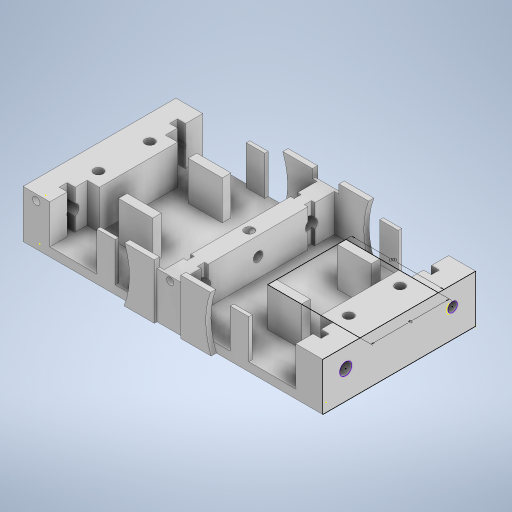
# Autodesk Inventor part: SCHOOL PROJECT
Saved by Autodesk Inventor 2024 (Build 280153000, 153)
## iProperties
Created: 2025-05-09
Part Number: SCHOOL PROJECT
Material: Generic
Document SubType Name: Modeling
Designer: arikm
Density: 1 g/cm^3
Appearance: Default
Author: arikm
Autodesk Inventor part; units mm, degrees
ref_plane "YZ Plane" through (0, 0, 0) normal (1, 0, 0) x (0, 1, 0)
ref_plane "XZ Plane" through (0, 0, 0) normal (0, 1, 0) x (-1, 0, 0)
ref_plane "XY Plane" through (0, 0, 0) normal (0, 0, 1) x (1, 0, 0)
sketch "Sketch1" plane through (0, 0, 0) normal (0, 1, 0) x (-1, 0, 0)
  line L0 (0, 0) -> (-70, 0)
  line L1 (-70, 0) -> (-70, -19.4)
  line L2 (-70, -19.4) -> (0, -19.4)
  line L3 (0, -19.4) -> (0, 0)
  line L4 (0, 0) -> (-4.4, 0)
  line L5 (-4.4, 0) -> (-4.4, -19.4)
  line L6 (-4.4, -19.4) -> (0, -19.4)
  line L7 (0, -19.4) -> (0, 0)
  line L8 (0, -9.7) -> (-4.4, -9.7)
  line L9 (0, -7.95) -> (-4.4, -7.95)
  line L10 (0, -11.45) -> (-4.4, -11.45)
  line L11 (5, -24.4) -> (-75, -24.4)
  line L12 (-75, -24.4) -> (-75, 5)
  line L13 (-75, 5) -> (5, 5)
  line L14 (5, 5) -> (5, -24.4)
  line L15 (-75, 0) -> (-75, 2)
  line L16 (-75, 2) -> (5, 2)
  dimension "d0" = 70
  dimension "d1" = 19.4
  dimension "d2" = 4.4
  dimension "d3" = 1.75
  dimension "d4" = 1.75
  dimension "d5" = 5
  dimension "d6" = 2
  constraints: 34 end point, 8 parallel, 4 perpendicular, 4 point on line, 2 horizontal, 2 midpoint, 3 other
  measures "d0" distance of L2.end L1.end
  measures "d1" distance of L1.end L0.end
  measures "d2" distance of L6.end L5.end
  measures "d3" distance between parallel lines of L8 L9
  measures "d4" distance between parallel lines of L8 L10
  measures "d5" distance between parallel lines of L2 L11
  measures "d6" distance of L15.start L15.end
extrude "Extrusion1" add sketch "Sketch1" along normal blind 22.4 contours L3 L9 L5 L0 | L3 L2 L5 L10 | L11 L12 L16 L14
sketch "Sketch2" plane through (0, 0, 0) normal (0, -1, 0) x (1, 0, 0)
  line L0 (-5, -24.4) -> (-5, 2) projected
  line L1 (75, -24.4) -> (-5, -24.4) projected
  line L2 (-5, 2) -> (75, 2)
  line L3 (75, 2) -> (75, -24.4)
  line L4 (75, -24.4) -> (-5, -24.4)
  line L5 (-5, -24.4) -> (-5, 2)
  point P0 (0, 0)
  constraints: 8 end point, 2 parallel, 1 horizontal, 1 perpendicular
extrude "Extrusion2" add sketch "Sketch2" along normal blind 1
sketch "Sketch3" plane through (0, 22.4, 0) normal (0, 1, 0) x (1, 0, 0)
  line L0 (75, -2) -> (75, 24.4) projected
  line L1 (75, 24.4) -> (48, 24.4)
  line L2 (48, 24.4) -> (48, -5.6)
  line L3 (48, -5.6) -> (75, -5.6)
  line L4 (75, -5.6) -> (75, 24.4)
  point P0 (0, 0)
  dimension "d11" = 27
  dimension "d12" = 30
  constraints: 8 end point, 2 parallel, 1 horizontal, 1 perpendicular
  measures "d11" distance of L3.end L2.end
  measures "d12" distance of L2.end L1.end
extrude "Extrusion3" cut sketch "Sketch3" against normal up to surface (22.4 mm away)
sketch "Sketch4" plane through (0, 22.4, 0) normal (0, 1, 0) x (1, 0, 0)
  line L0 (48, 0) -> (4.4, 0) projected
  line L1 (4.4, 0) -> (13.4, 0)
  line L2 (13.4, 0) -> (12.4, 0)
  line L3 (12.4, 0) -> (17.4, 0)
  line L4 (17.4, 0) -> (12.4, 0)
  line L5 (12.4, 0) -> (12.4, -8.176)
  line L6 (12.4, -8.176) -> (17.4, -8.176)
  line L7 (17.4, -8.176) -> (17.4, 0)
  line L8 (12.4, -8.176) -> (17.4, -8.176)
  line L9 (17.4, -8.176) -> (17.4, 29.1171)
  line L10 (17.4, 29.1171) -> (12.4, 29.1171)
  line L11 (12.4, 29.1171) -> (12.4, -8.176)
  point P0 (0, 0)
  dimension "d15" = 9
  dimension "d16" = 1
  dimension "d17" = 5
  constraints: 22 end point, 4 parallel, 4 point on line, 2 horizontal, 2 perpendicular
  measures "d15" distance of L0.end L1.end
  measures "d16" distance of L1.end L2.end
  measures "d17" distance of L2.end L3.end
extrude "Extrusion4" cut sketch "Sketch4" against normal up to surface (22.4 mm away)
sketch "Sketch5" plane through (-5, -1, 2) normal (0, 0, 1) x (1, 0, 0)
  line L0 (17.4, 1) -> (22.4, 1) projected
  line L1 (53, 23.4) -> (22.4, 23.4) projected
  line L2 (17.4, 1) -> (27.4, 1)
  line L3 (27.4, 1) -> (27.4, 23.4)
  line L4 (27.4, 23.4) -> (17.4, 23.4)
  line L5 (17.4, 23.4) -> (17.4, 1)
  point P0 (5, 1)
  dimension "d20" = 10
  constraints: 8 end point, 2 parallel, 1 horizontal, 1 perpendicular, 1 point on line
  measures "d20" distance of L4.end L3.end
extrude "Extrusion5" cut sketch "Sketch5" against normal through all
sketch "Sketch6" plane through (-5, -1, 2) normal (0, 0, 1) x (1, 0, 0)
  line L0 (17.4, 23.4) -> (17.4, 1) projected
  line L1 (17.4, 23.4) -> (9.4, 23.4)
  line L2 (17.4, 23.4) -> (0, 23.4) projected
  line L3 (53, 23.4) -> (27.4, 23.4) projected
  line L4 (27.4, 23.4) -> (35.4, 23.4)
  line L5 (9.4, 23.4) -> (35.4, 23.4)
  line L6 (35.4, 23.4) -> (35.4, 1)
  line L7 (35.4, 1) -> (9.4, 1)
  line L8 (9.4, 1) -> (9.4, 23.4)
  point P0 (5, 1)
  dimension "d23" = 8
  dimension "d24" = 8
  constraints: 12 end point, 2 parallel, 2 point on line, 1 horizontal, 1 perpendicular
  measures "d23" distance of L0.start L1.end
  measures "d24" distance of L3.end L4.end
extrude "Extrusion6" cut sketch "Sketch6" against normal blind 10
sketch "Sketch7" plane through (0, 0, 0) normal (0, 1, 0) x (1, 0, 0)
  line L0 (-5, 24.4) -> (75, 24.4) projected
  line L1 (75, 24.4) -> (75, 59.4)
  line L2 (75, -2) -> (-5, -2) projected
  line L3 (75, -2) -> (-5, -2)
  line L4 (-5, -2) -> (-5, 24.4)
  line L5 (-5, 24.4) -> (75, 24.4)
  line L6 (75, 24.4) -> (75, -2)
  line L7 (4.4, -2) -> (4.4, 7.95) projected
  line L8 (4.4, 7.95) -> (4.4, -2)
  line L9 (4.4, 7.95) -> (0, 7.95)
  line L10 (0, 7.95) -> (0, 11.45) projected
  line L11 (0, 7.95) -> (0, 11.45)
  line L12 (0, 11.45) -> (4.4, 11.45)
  line L13 (4.4, 11.45) -> (4.4, 19.4) projected
  line L14 (0, 11.45) -> (4.4, 11.45)
  line L15 (4.4, 11.45) -> (4.4, 19.4)
  line L16 (12.4, 19.4) -> (12.4, 24.4) projected
  line L17 (4.4, 19.4) -> (12.4, 19.4)
  line L18 (12.4, 19.4) -> (12.4, 24.4)
  line L19 (22.4, 19.4) -> (22.4, 24.4) projected
  line L20 (12.4, 24.4) -> (22.4, 24.4)
  line L21 (22.4, 19.4) -> (48, 19.4) projected
  line L22 (22.4, 24.4) -> (48, 24.4)
  line L23 (48, 24.4) -> (48, 19.4)
  line L24 (48, 19.4) -> (22.4, 19.4)
  line L25 (22.4, 19.4) -> (22.4, 24.4)
  line L26 (75, 41.9) -> (-5, 41.9)
  line L27 (48, 0) -> (30.4, 0) projected
  line L28 (30.4, -2) -> (48, -2)
  line L29 (48, -2) -> (48, 0)
  line L30 (48, 0) -> (30.4, 0)
  line L31 (30.4, 0) -> (30.4, -2)
  line L32 (-5, 59.4) -> (75, 59.4)
  line L33 (75, 85.8) -> (-5, 85.8)
  line L34 (-5, 85.8) -> (-5, 59.4)
  line L35 (75, 59.4) -> (75, 85.8)
  line L36 (4.4, 75.85) -> (4.4, 85.8)
  line L37 (4.4, 75.85) -> (0, 75.85)
  line L38 (0, 75.85) -> (0, 72.35)
  line L39 (0, 72.35) -> (4.4, 72.35)
  line L40 (4.4, 72.35) -> (4.4, 64.4)
  line L41 (12.4, 64.4) -> (12.4, 59.4)
  line L42 (4.4, 64.4) -> (12.4, 64.4)
  line L43 (22.4, 64.4) -> (22.4, 59.4)
  line L44 (48, 59.4) -> (48, 64.4)
  line L45 (48, 64.4) -> (22.4, 64.4)
  line L46 (48, 83.8) -> (30.4, 83.8)
  line L47 (48, 85.8) -> (48, 83.8)
  line L48 (30.4, 83.8) -> (30.4, 85.8)
  point P0 (0, 0)
  dimension "d27" = 35
  constraints: 80 end point, 24 symmetric about line, 7 perpendicular, 6 parallel, 5 horizontal, 4 collinear, 1 midpoint, 1 point on line, 1 vertical
  measures "d27" distance of L0.end L1.end
extrude "Extrusion7" add sketch "Sketch7" against normal blind 1 contours L34 L33 L36 L37 L38 L39 L40 L42 L41 L32 | L41 L42 L40 L39 L38 L37 L36 L33 L48 L46 L47 L35 L32 L44 L45 L43 | L43 L45 L44 L32 | L33 L47 L46 L48
extrude "Extrusion8" add sketch "Sketch7" along normal up to surface (22.4 mm away) contours L34 L33 L36 L37 L38 L39 L40 L42 L41 L32 | L43 L45 L44 L32 | L33 L47 L46 L48
thicken "Thicken1" operation cut thickness 1 both sides no extend neighbours no toward (1, 0, 0) faces at (30.4, 7.4667, 0.6667)
thicken "Thicken2" operation cut thickness 1 both sides no extend neighbours no toward (1, 0, 0) faces at (30.4, 7.4667, -85.1333)
thicken "Thicken3" operation cut thickness 1 both sides no extend neighbours no toward (-1, 0, 0) faces at (12.4, 7.4667, -22.7333)
thicken "Thicken4" operation cut thickness 1 both sides no extend neighbours no toward (-1, 0, 0) faces at (12.4, 7.4667, -61.0667)
thicken "Thicken7" operation cut thickness 0.2 both sides no extend neighbours no toward (-1, 0, 0) faces at (0, 7.4667, -9.1167)
thicken "Thicken8" operation cut thickness 0.2 both sides no extend neighbours no toward (-1, 0, 0) faces at (0, 7.4667, -73.5167)
sketch "Sketch8" plane through (0, 22.4, 0) normal (0, 1, 0) x (1, 0, 0)
  line L0 (48, 0) -> (48, -2) projected
  line L1 (-5, 85.8) -> (75, 85.8) projected
  line L2 (48, -2) -> (42, -2)
  line L3 (42, -2) -> (42, 85.8)
  line L4 (42, 85.8) -> (48, 85.8)
  line L5 (48, 85.8) -> (48, -2)
  point P0 (0, 0)
  dimension "d48" = 6
  constraints: 8 end point, 2 parallel, 1 horizontal, 1 perpendicular, 1 point on line
  measures "d48" distance of L3.end L4.end
extrude "Extrusion9" cut sketch "Sketch8" against normal up to surface (22.4 mm away)
sketch "Sketch9" plane through (0, 0, 0) normal (0, 1, 0) x (1, 0, 0)
  line L0 (75, 24.4) -> (75, -2) projected
  line L1 (-5, 24.4) -> (75, 24.4) projected
  line L2 (75, -2) -> (70, -2)
  line L3 (70, -2) -> (70, 24.4)
  line L4 (70, 24.4) -> (75, 24.4)
  line L5 (75, 24.4) -> (75, -2)
  line L6 (75, 59.4) -> (75, 85.8) projected
  line L7 (-5, 85.8) -> (75, 85.8) projected
  line L8 (75, 59.4) -> (70, 59.4)
  line L9 (70, 59.4) -> (70, 85.8)
  line L10 (70, 85.8) -> (75, 85.8)
  line L11 (75, 85.8) -> (75, 59.4)
  point P0 (0, 0)
  dimension "d51" = 5
  dimension "d52" = 5
  constraints: 16 end point, 4 parallel, 2 horizontal, 2 perpendicular, 2 point on line
  measures "d51" distance of L3.end L4.end
  measures "d52" distance of L9.end L10.end
extrude "Extrusion10" add sketch "Sketch9" along normal up to surface (22.4 mm away)
sketch "Sketch10" plane through (75, -1, 2) normal (1, 0, 0) x (0, 0, -1)
  line L0 (2, 1) -> (0, 1) projected
  line L1 (26.4, 23.4) -> (26.4, 1) projected
  line L2 (0, 1) -> (26.4, 1)
  line L3 (26.4, 1) -> (26.4, 23.4)
  line L4 (26.4, 23.4) -> (0, 23.4)
  line L5 (0, 23.4) -> (0, 1)
  line L6 (0, 12.2) -> (87.8, 12.2)
  line L7 (87.8, 1) -> (87.8, 23.4) projected
  line L8 (61.4, 0) -> (61.4, 23.4) projected
  line L9 (61.4, 12.2) -> (87.8, 12.2)
  circle A0 centre (13.2, 12.2) radius 3.5
  circle A1 centre (74.6, 12.2) radius 3.5
  dimension "d55" = 7
  dimension "d56" = 7
  constraints: 12 end point, 3 midpoint, 3 point on line, 2 centre point, 2 parallel, 1 collinear, 1 horizontal, 1 perpendicular
  measures "d55" diameter of A0
  measures "d56" diameter of A1
extrude "Extrusion11" cut sketch "Sketch10" against normal through all contours A0 L6 | L6 A0 | A1 L6 | L6 A1
sketch "Sketch11" plane through (70, 22.4, 2) normal (0, 1, 0) x (1, 0, 0)
  line L0 (0, 0) -> (0, 26.4) projected
  line L1 (0, 13.2) -> (2, 13.2)
  line L2 (0, 13.2) -> (2, 13.2) construction
  line L3 (2, 13.2) -> (0, 13.2)
  line L4 (0, 13.2) -> (0, 11.2)
  line L5 (0, 11.2) -> (2, 11.2)
  line L6 (2, 11.2) -> (2, 13.2)
  line L7 (0, 11.2) -> (2, 11.2)
  line L8 (2, 11.2) -> (2, 15.2)
  line L9 (2, 15.2) -> (0, 15.2)
  line L10 (0, 15.2) -> (0, 11.2)
  line L11 (0, 61.4) -> (0, 87.8) projected
  line L12 (0, 74.6) -> (2, 74.6)
  line L13 (2, 74.6) -> (2, 73.4639)
  line L14 (2, 73.4639) -> (0, 73.4639)
  line L15 (0, 73.4639) -> (0, 74.6)
  line L16 (2, 74.6) -> (0, 74.6)
  line L17 (0, 74.6) -> (0, 76.6)
  line L18 (0, 76.6) -> (2, 76.6)
  line L19 (2, 76.6) -> (2, 74.6)
  line L20 (0, 74.6) -> (2, 74.6)
  line L21 (2, 74.6) -> (2, 72.6)
  line L22 (2, 72.6) -> (0, 72.6)
  line L23 (0, 72.6) -> (0, 74.6)
  point P0 (-70, 2)
  point P1 (2, 13.2)
  point P2 (0, 15.2)
  point P3 (2, 73.4639)
  dimension "d59" = 2
  dimension "d60" = 0
  dimension "d61" = 2
  dimension "d62" = 4
  dimension "d63" = 2
  dimension "d64" = 2
  dimension "d65" = 2
  constraints: 44 end point, 10 parallel, 7 horizontal, 5 perpendicular, 4 point on line, 2 midpoint, 1 collinear
  measures "d59" distance of L1.start L1.end
  measures "d60" distance between parallel lines of L1 L2
  measures "d61" distance of L4.end L3.end
  measures "d62" distance of L8.end L7.end
  measures "d63" distance of L13.end L14.end
  measures "d64" distance of L16.end L17.end
  measures "d65" distance of L20.end L21.end
extrude "Extrusion12" cut sketch "Sketch11" against normal up to surface contours L0 L1 L6 L5 | L0 L9 L8 L1 round surface about axis through (75, 11.2, -11.2) along (-1, 0, 0) radius 3.5 far side no
extrude "Extrusion13" cut sketch "Sketch11" against normal up to surface contours L11 L14 L21 L22 | L11 L12 L13 L14 | L11 L18 L19 L12 round surface about axis through (75, 11.2, -72.6) along (-1, 0, 0) radius 3.5 far side no
sketch "Sketch12" plane through (0, 22.4, 0) normal (0, 1, 0) x (1, 0, 0)
  line L0 (4.4, 14.7) -> (4.4, 11.45) projected
  line L1 (-0.2, 11.45) -> (4.4, 11.45)
  line L2 (4.4, 11.45) -> (4.4, 12.45)
  line L3 (4.4, 12.45) -> (-0.2, 12.45)
  line L4 (-0.2, 12.45) -> (-0.2, 11.45)
  point P0 (0, 0)
  dimension "d70" = 1
  constraints: 8 end point, 2 parallel, 1 horizontal, 1 perpendicular, 1 point on line
  measures "d70" distance of L2.end L1.end
extrude "Extrusion14" cut sketch "Sketch12" against normal up to surface (22.4 mm away)
sketch "Sketch13" plane through (-5, 22.4, -85.8) normal (0, 1, 0) x (1, 0, 0)
  line L0 (9.4, -13.45) -> (9.4, -21.4) projected
  line L1 (9.4, -13.45) -> (4.8, -13.45)
  line L2 (4.8, -13.45) -> (4.8, -14.45)
  line L3 (4.8, -14.45) -> (9.4, -14.45)
  line L4 (9.4, -14.45) -> (9.4, -13.45)
  point P0 (5, -85.8)
  point P1 (9.4, -14.45)
  dimension "d73" = 1
  constraints: 8 end point, 2 parallel, 1 horizontal, 1 perpendicular
  measures "d73" distance of L2.end L1.end
extrude "Extrusion15" cut sketch "Sketch13" against normal up to surface (22.4 mm away)
sketch "Sketch14" plane through (0, 0, 0) normal (0, 1, 0) x (1, 0, 0)
  line L0 (11.4, 24.4) -> (-5, 24.4) projected
  line L1 (75, 59.4) -> (-5, 59.4) projected
  line L2 (-5, 24.4) -> (75, 24.4)
  line L3 (75, 24.4) -> (75, 59.4)
  line L4 (75, 59.4) -> (-5, 59.4)
  line L5 (-5, 59.4) -> (-5, 24.4)
  point P0 (0, 0)
  constraints: 8 end point, 2 parallel, 1 horizontal, 1 perpendicular
extrude "Extrusion16" add sketch "Sketch14" against normal up to surface (1 mm away)
sketch "Sketch15" plane through (0, 0, 0) normal (0, 1, 0) x (1, 0, 0)
  line L0 (-5, -2) -> (-5, 85.8) projected
  line L1 (75, 85.8) -> (75, -2) projected
  line L2 (-5, -2) -> (75, -2)
  line L3 (75, -2) -> (75, 85.8)
  line L4 (75, 85.8) -> (-5, 85.8)
  line L5 (-5, 85.8) -> (-5, -2)
  line L6 (-0.2, 7.95) -> (-0.2, 12.45) projected
  line L7 (-0.2, 12.45) -> (4.4, 12.45) projected
  line L8 (-0.2, 7.95) -> (4.4, 7.95)
  line L9 (4.4, 7.95) -> (4.4, 12.45)
  line L10 (4.4, 12.45) -> (-0.2, 12.45)
  line L11 (-0.2, 12.45) -> (-0.2, 7.95)
  line L12 (11.4, 24.4) -> (-5, 24.4) projected
  line L13 (4.4, 19.4) -> (11.4, 19.4) projected
  line L14 (-5, 24.4) -> (11.4, 24.4)
  line L15 (11.4, 24.4) -> (11.4, 19.4)
  line L16 (11.4, 19.4) -> (-5, 19.4)
  line L17 (-5, 19.4) -> (-5, 24.4)
  line L18 (-5, -2) -> (4.4, -2)
  line L19 (4.4, -2) -> (4.4, 19.4)
  line L20 (4.4, 19.4) -> (-5, 19.4)
  line L21 (-5, 19.4) -> (-5, -2)
  line L22 (11.4, 19.4) -> (-5, 19.4)
  line L23 (-5, 19.4) -> (-5, 24.4)
  line L24 (-5, 24.4) -> (11.4, 24.4)
  line L25 (11.4, 24.4) -> (11.4, 19.4)
  line L26 (31.4, -2) -> (31.4, 0) projected
  line L27 (42, 0) -> (31.4, 0) projected
  line L28 (31.4, -2) -> (42, -2)
  line L29 (42, -2) -> (42, 0)
  line L30 (42, 0) -> (31.4, 0)
  line L31 (31.4, 0) -> (31.4, -2)
  line L32 (22.4, 24.4) -> (22.4, 19.4) projected
  line L33 (22.4, 19.4) -> (42, 19.4)
  line L34 (42, 19.4) -> (42, 24.4)
  line L35 (42, 24.4) -> (22.4, 24.4)
  line L36 (22.4, 24.4) -> (22.4, 19.4)
  line L37 (70, 13.2) -> (70, 24.4) projected
  line L38 (75, -2) -> (70, -2)
  line L39 (70, -2) -> (70, 24.4)
  line L40 (70, 24.4) -> (75, 24.4)
  line L41 (75, 24.4) -> (75, -2)
  line L42 (70, 9.2) -> (72, 9.2) projected
  line L43 (72, 13.2) -> (70, 13.2) projected
  line L44 (70, 9.2) -> (72, 9.2)
  line L45 (72, 9.2) -> (72, 13.2)
  line L46 (72, 13.2) -> (70, 13.2)
  line L47 (70, 13.2) -> (70, 9.2)
  line L48 (-5, 59.4) -> (-5, 24.4) projected
  line L49 (-5, 41.9) -> (75, 41.9)
  line L50 (-5, 85.8) -> (-5, -2)
  line L51 (75, -2) -> (75, 85.8)
  line L52 (-5, 85.8) -> (75, 85.8)
  line L53 (-0.2, 75.85) -> (-0.2, 71.35)
  line L54 (-0.2, 71.35) -> (4.4, 71.35)
  line L55 (-0.2, 75.85) -> (4.4, 75.85)
  line L56 (4.4, 75.85) -> (4.4, 71.35)
  line L57 (4.4, 64.4) -> (11.4, 64.4)
  line L58 (-5, 59.4) -> (11.4, 59.4)
  line L59 (4.4, 85.8) -> (4.4, 64.4)
  line L60 (11.4, 59.4) -> (11.4, 64.4)
  line L61 (31.4, 85.8) -> (31.4, 83.8)
  line L62 (42, 83.8) -> (31.4, 83.8)
  line L63 (42, 85.8) -> (42, 83.8)
  line L64 (70, 85.8) -> (70, 59.4)
  line L65 (70, 59.4) -> (75, 59.4)
  line L66 (70, 74.6) -> (72, 74.6)
  line L67 (72, 70.6) -> (70, 70.6)
  line L68 (72, 74.6) -> (72, 70.6)
  line L69 (155, -2) -> (155, 85.8)
  line L70 (155, -2) -> (75, -2)
  line L71 (75, 85.8) -> (155, 85.8)
  line L72 (150.2, 7.95) -> (150.2, 12.45)
  line L73 (150.2, 12.45) -> (145.6, 12.45)
  line L74 (150.2, 7.95) -> (145.6, 7.95)
  line L75 (138.6, 24.4) -> (155, 24.4)
  line L76 (145.6, 19.4) -> (138.6, 19.4)
  line L77 (138.6, 24.4) -> (138.6, 19.4)
  line L78 (145.6, -2) -> (145.6, 19.4)
  line L79 (155, 19.4) -> (155, -2)
  line L80 (118.6, -2) -> (118.6, 0)
  line L81 (108, -2) -> (108, 0)
  line L82 (108, 0) -> (118.6, 0)
  line L83 (127.6, 24.4) -> (127.6, 19.4)
  line L84 (127.6, 19.4) -> (108, 19.4)
  line L85 (108, 19.4) -> (108, 24.4)
  line L86 (108, 24.4) -> (127.6, 24.4)
  line L87 (80, -2) -> (80, 24.4)
  line L88 (80, 24.4) -> (75, 24.4)
  line L89 (80, 9.2) -> (78, 9.2)
  line L90 (78, 13.2) -> (80, 13.2)
  line L91 (78, 9.2) -> (78, 13.2)
  line L92 (150.2, 75.85) -> (145.6, 75.85)
  line L93 (150.2, 75.85) -> (150.2, 71.35)
  line L94 (150.2, 71.35) -> (145.6, 71.35)
  line L95 (145.6, 75.85) -> (145.6, 71.35)
  line L96 (145.6, 85.8) -> (145.6, 64.4)
  line L97 (155, 59.4) -> (138.6, 59.4)
  line L98 (138.6, 59.4) -> (138.6, 64.4)
  line L99 (145.6, 64.4) -> (138.6, 64.4)
  line L100 (108, 83.8) -> (118.6, 83.8)
  line L101 (108, 85.8) -> (108, 83.8)
  line L102 (118.6, 85.8) -> (118.6, 83.8)
  line L103 (80, 85.8) -> (80, 59.4)
  line L104 (80, 59.4) -> (75, 59.4)
  line L105 (78, 74.6) -> (78, 70.6)
  line L106 (80, 74.6) -> (78, 74.6)
  line L107 (78, 70.6) -> (80, 70.6)
  line L108 (155, 41.9) -> (75, 41.9)
  line L109 (127.6, 19.4) -> (108, 19.4)
  line L110 (108, 19.4) -> (108, 24.4)
  line L111 (108, 24.4) -> (127.6, 24.4)
  line L112 (127.6, 24.4) -> (127.6, 19.4)
  line L113 (127.6, 19.4) -> (108, 19.4)
  line L114 (108, 19.4) -> (108, 24.4)
  line L115 (108, 24.4) -> (127.6, 24.4)
  line L116 (127.6, 24.4) -> (127.6, 19.4)
  line L117 (108, 64.4) -> (108, 59.4)
  line L118 (127.6, 64.4) -> (108, 64.4)
  line L119 (127.6, 59.4) -> (127.6, 64.4)
  line L120 (108, 59.4) -> (127.6, 59.4)
  point P0 (0, 0)
  point P1 (75, -2)
  constraints: 216 end point, 86 symmetric about line, 22 parallel, 12 horizontal, 11 perpendicular, 4 point on line, 3 midpoint
extrude "Extrusion17" add sketch "Sketch15" against normal blind 1 contours L108 L69 L75 L77 L76 L78 L70 L80 L82 L81 L87 L88 L1 | L1 L104 L103 L71 L101 L100 L102 L96 L95 L99 L98 L97 L69 L108 | L1 L71 L103 L106 L105 L107 L104 | L88 L87 L90 L91 L89 L70 L1 | L69 L70 L78 L74 L72 L73 L76 L77 L75 | L97 L98 L99 L96 L94 L93 L92 L71 L69 | L107 L105 L106 L103 | L87 L89 L91 L90 | L81 L82 L80 L70 | L71 L102 L100 L101 | L92 L93 L94 L95 | L78 L73 L72 L74 | L83 L84 L85 L86 | L118 L119 L120 L117
extrude "Extrusion18" add sketch "Sketch15" along normal up to surface (22.4 mm away) contours L1 L71 L103 L106 L105 L107 L104 | L88 L87 L90 L91 L89 L70 L1 | L69 L70 L78 L74 L72 L73 L76 L77 L75 | L97 L98 L99 L96 L94 L93 L92 L71 L69 | L81 L82 L80 L70 | L71 L102 L100 L101 | L83 L84 L85 L86 | L118 L119 L120 L117
sketch "Sketch16" plane through (-5, 22.4, -24.4) normal (-1, 0, 0) x (0, 0, 1)
  arc A0 (-51.45, -9.901) -> (-51.45, -12.499) centre (-48.2, -11.2) ccw projected
  circle A1 centre (-48.2, -11.2) radius 3.5
  circle A2 centre (13.2, -11.2) radius 3.5 projected
  circle A3 centre (13.2, -11.2) radius 3.5
  point P0 (24.4, -22.4)
  constraints: 2 centre point, 2 coincident
extrude "Extrusion19" add sketch "Sketch16" against normal through all
extrude "Extrusion20" cut sketch "Sketch16" against normal through all
sketch "Sketch17" plane through (0, -1, 0) normal (0, -1, 0) x (1, 0, 0)
  line L0 (-5, -85.8) -> (155, -85.8) projected
  line L1 (155, 2) -> (-5, 2)
  line L2 (-5, 2) -> (-5, -85.8)
  line L3 (-5, -85.8) -> (155, -85.8)
  line L4 (155, -85.8) -> (155, 2)
  point P0 (0, 0)
  constraints: 8 end point, 2 parallel, 1 horizontal, 1 perpendicular
extrude "Extrusion21" add sketch "Sketch17" along normal blind 4
sketch "Sketch18" plane through (0, 0, 0) normal (0, 1, 0) x (1, 0, 0)
  line L0 (22.4, 59.4) -> (42, 59.4) projected
  line L1 (32.2, 59.4) -> (32.2, 24.4)
  line L2 (42, 24.4) -> (22.4, 24.4) projected
  line L3 (108, 24.4) -> (127.6, 24.4) projected
  line L4 (117.8, 24.4) -> (117.8, 59.4)
  line L5 (127.6, 59.4) -> (108, 59.4) projected
  line L6 (80, 24.4) -> (70, 24.4) projected
  line L7 (75, 24.4) -> (75, 59.4)
  line L8 (80, 59.4) -> (70, 59.4) projected
  circle A0 centre (32.2, 41.9) radius 3.25
  circle A1 centre (75, 41.9) radius 3.25
  circle A2 centre (117.8, 41.9) radius 3.25
  point P0 (0, 0)
  dimension "d88" = 6.5
  dimension "d89" = 6.5
  dimension "d90" = 6.5
  constraints: 9 midpoint, 6 end point, 3 centre point
  measures "d88" diameter of A0
  measures "d89" diameter of A1
  measures "d90" diameter of A2
extrude "Extrusion22" cut sketch "Sketch18" against normal through all
sketch "Sketch19" plane through (0, 0, 0) normal (0, 1, 0) x (1, 0, 0)
  circle A0 centre (32.2, 41.9) radius 3.25 projected
  circle A1 centre (32.2, 41.9) radius 5
  circle A2 centre (75, 41.9) radius 3.25 projected
  circle A3 centre (75, 41.9) radius 5
  circle A4 centre (117.8, 41.9) radius 3.25 projected
  circle A5 centre (117.8, 41.9) radius 5
  point P0 (0, 0)
  dimension "d93" = 10
  dimension "d94" = 10
  dimension "d95" = 10
  constraints: 3 centre point, 3 coincident
  measures "d93" diameter of A1
  measures "d94" diameter of A3
  measures "d95" diameter of A5
extrude "Extrusion23" cut sketch "Sketch19" against normal blind 3 contours A0 | A1 | A2 | A3 | A4 | A5
sketch "Sketch20" plane through (0, 0, 0) normal (0, 1, 0) x (1, 0, 0)
  circle A0 centre (75, 41.9) radius 5 projected
  circle A1 centre (75, 41.9) radius 100
  line L0 (138.6, 24.4) -> (155, 24.4) projected
  line L1 (146.8, 24.4) -> (146.8, 59.4)
  line L2 (155, 59.4) -> (138.6, 59.4) projected
  line L3 (155, 59.4) -> (138.6, 59.4)
  line L4 (138.6, 59.4) -> (138.6, 24.4)
  line L5 (138.6, 24.4) -> (155, 24.4)
  line L6 (155, 24.4) -> (155, 59.4)
  line L7 (-5, -2) -> (-5, 85.8) projected
  line L8 (11.4, 64.4) -> (11.4, 59.4) projected
  line L9 (-5, 24.4) -> (11.4, 24.4)
  line L10 (11.4, 24.4) -> (11.4, 59.4)
  line L11 (11.4, 59.4) -> (-5, 59.4)
  line L12 (-5, 59.4) -> (-5, 24.4)
  point P0 (0, 0)
  constraints: 18 end point, 4 parallel, 2 horizontal, 2 midpoint, 2 perpendicular, 1 centre point, 1 coincident, 1 point on line
extrude "Extrusion24" add sketch "Sketch20" along normal up to surface (22.4 mm away) contours L4 L2 L1 L0 | L1 L2 L6 L0 | L7 L11 L10 L9
sketch "Sketch21" plane through (0, 0, 0) normal (0, 1, 0) x (1, 0, 0)
  line L0 (67.8253, 32.1607) -> (82.8688, 32.1607)
  line L1 (82.8688, 32.1607) -> (82.8688, 49.81)
  line L2 (82.8688, 49.81) -> (67.8253, 49.81)
  line L3 (67.8253, 49.81) -> (67.8253, 32.1607)
  point P0 (0, 0)
  constraints: 8 end point, 2 parallel, 1 horizontal, 1 perpendicular
extrude "Extrusion25" add sketch "Sketch21" against normal up to surface (5 mm away)
sketch "Sketch22" plane through (0, 0, 0) normal (0, 1, 0) x (1, 0, 0)
  line L0 (70, -2) -> (70, 24.4) projected
  line L1 (80, 70.6) -> (80, 59.4) projected
  line L2 (70, 24.4) -> (80, 24.4)
  line L3 (80, 24.4) -> (80, 59.4)
  line L4 (80, 59.4) -> (70, 59.4)
  line L5 (70, 59.4) -> (70, 24.4)
  point P0 (0, 0)
  constraints: 8 end point, 2 parallel, 1 horizontal, 1 perpendicular
extrude "Extrusion26" add sketch "Sketch22" along normal up to surface (22.4 mm away)
sketch "Sketch23" plane through (70, 22.4, 2) normal (0, 1, 0) x (1, 0, 0)
  line L0 (0, 15.2) -> (0, 72.6) projected
  line L1 (0, 43.9) -> (10, 43.9)
  line L2 (10, 72.6) -> (10, 15.2) projected
  circle A0 centre (5, 43.9) radius 2.7
  line L3 (68.7195, 43.9) -> (85, 43.9)
  line L4 (85, 87.8) -> (85, 0) projected
  line L5 (76.8598, 43.9) -> (76.8598, 14.45)
  line L6 (80.2, 14.45) -> (75.6, 14.45) projected
  line L7 (76.8598, 43.9) -> (76.8598, 73.35)
  line L8 (75.6, 73.35) -> (80.2, 73.35) projected
  line L9 (5, 43.9) -> (5, 33.1975)
  line L10 (-66.8598, 43.9) -> (-66.8598, 14.45)
  line L11 (-66.8598, 43.9) -> (-66.8598, 73.35)
  line L12 (-66.8598, 43.9) -> (-66.8598, 14.45)
  circle A1 centre (-66.8598, 29.175) radius 2.7
  circle A2 centre (-66.8598, 58.625) radius 2.7
  circle A3 centre (76.8598, 29.175) radius 2.7
  circle A4 centre (76.8598, 58.625) radius 2.7
  point P0 (-70, 2)
  dimension "d15" = 9
  dimension "d105" = 5.4
  dimension "d106" = 5.4
  dimension "d107" = 5.4
  dimension "d108" = 5.4
  dimension "d109" = 5.4
  constraints: 16 end point, 9 midpoint, 5 centre point, 5 point on line, 3 symmetric about line, 2 vertical, 1 collinear
  measures "d105" diameter of A0
  measures "d106" diameter of A1
  measures "d107" diameter of A2
  measures "d108" diameter of A3
  measures "d109" diameter of A4
extrude "Extrusion27" cut sketch "Sketch23" against normal blind 6
sketch "Sketch25" plane through (155, 22.4, 2) normal (1, 0, 0) x (0, 0, -1)
  line L0 (0, 0) -> (0, -22.4) projected
  line L1 (87.8, -27.4) -> (87.8, 0) projected
  line L2 (0, 0) -> (87.8, 0)
  line L3 (87.8, 0) -> (87.8, -27.4)
  line L4 (87.8, -27.4) -> (0, -27.4)
  line L5 (0, -27.4) -> (0, 0)
  line L6 (0, 0) -> (87.8, 0)
  line L7 (87.8, 0) -> (87.8, -27.4)
  line L8 (87.8, -27.4) -> (0, -27.4)
  line L9 (0, -27.4) -> (0, 0)
  circle A0 centre (13.2, -11.2) radius 3.5 projected
  circle A1 centre (13.2, -11.2) radius 2.8
  arc A2 (76.6, -8.3277) -> (72.6, -8.3277) centre (74.6, -11.2) ccw projected
  circle A3 centre (74.6, -11.2) radius 2.8
  point P0 (2, -22.4)
  dimension "d112" = 5.6
  dimension "d113" = 5.6
  constraints: 16 end point, 4 parallel, 2 centre point, 2 coincident, 2 horizontal, 2 perpendicular
  measures "d112" diameter of A1
  measures "d113" diameter of A3
extrude "Extrusion28" add sketch "Sketch25" along normal blind 6 contours L2 L1 L4 L5 L0
sketch "Sketch26" plane through (-5, 22.4, -85.8) normal (-1, 0, 0) x (0, 0, 1)
  line L0 (87.8, -27.4) -> (87.8, 0) projected
  line L1 (0, -22.4) -> (0, 0) projected
  line L2 (87.8, -27.4) -> (0, -27.4)
  line L3 (0, -27.4) -> (0, 0)
  line L4 (0, 0) -> (87.8, 0)
  line L5 (87.8, 0) -> (87.8, -27.4)
  arc A0 (72.6, -8.3277) -> (76.6, -8.3277) centre (74.6, -11.2) ccw projected
  circle A1 centre (74.6, -11.2) radius 2.7
  arc A2 (9.95, -12.499) -> (14.45, -14.4692) centre (13.2, -11.2) ccw projected
  circle A3 centre (13.2, -11.2) radius 2.7
  point P0 (85.8, -22.4)
  dimension "d116" = 5.4
  dimension "d117" = 5.4
  constraints: 8 end point, 2 centre point, 2 coincident, 2 parallel, 1 horizontal, 1 perpendicular
  measures "d116" diameter of A1
  measures "d117" diameter of A3
extrude "Extrusion29" add sketch "Sketch26" along normal blind 6
sketch "Sketch27" plane through (0, 0, 0) normal (0, 1, 0) x (1, 0, 0)
  point P0 (0, 0)
sketch "Sketch28" plane through (161, 22.4, 2) normal (1, 0, 0) x (0, 0, -1)
  line L0 (87.8, 0) -> (0, 0) projected
  line L1 (0, 0) -> (87.8, 0)
  line L2 (87.8, 0) -> (87.8, -27.4)
  line L3 (87.8, -27.4) -> (0, -27.4)
  line L4 (0, -27.4) -> (0, 0)
  arc A0 (14.45, -7.9308) -> (9.95, -9.901) centre (13.2, -11.2) ccw projected
  circle A1 centre (13.2, -11.2) radius 3.5
  arc A2 (72.6, -8.3277) -> (72.6, -14.0723) centre (74.6, -11.2) ccw projected
  circle A3 centre (74.6, -11.2) radius 2.7
  point P0 (2, -22.4)
  constraints: 8 end point, 2 centre point, 2 coincident, 2 parallel, 1 horizontal, 1 perpendicular
sketch "Sketch29" plane through (0, 0, 0) normal (0, 1, 0) x (1, 0, 0)
  circle A0 centre (32.2, 41.9) radius 3.25 projected
  circle A1 centre (32.2, 41.9) radius 5
  circle A2 centre (117.8, 41.9) radius 3.25 projected
  circle A3 centre (117.8, 41.9) radius 5
  point P0 (0, 0)
  constraints: 2 centre point, 2 coincident
extrude "Extrusion30" add sketch "Sketch29" against normal up to surface (5 mm away) contours A0 | A1 | A2 | A3
sketch "Sketch30" plane through (4.4, 0, 2) normal (0, 0, 1) x (1, 0, 0)
  line L0 (-15.4, -5) -> (156.6, -5) projected
  line L1 (18, 0) -> (18, 22.4) projected
  line L2 (18, 11.2) -> (7, 11.2)
  line L3 (7, 0) -> (7, 22.4) projected
  line L4 (-15.4, -5) -> (-15.4, 11.2)
  line L5 (-15.4, 8.5) -> (-15.4, 13.9) projected
  line L6 (-15.4, 11.2) -> (156.6, 11.2)
  line L7 (-15.4, 11.2) -> (5.1, 11.2)
  line L8 (156.6, 11.2) -> (136.1, 11.2)
  circle A0 centre (5.1, 11.2) radius 33
  circle A1 centre (136.1, 11.2) radius 33
  line L9 (70.6, -5) -> (45.6, -5)
  line L10 (45.6, -5) -> (95.6, -5)
  circle A2 centre (5.1, 11.2) radius 43.6198
  circle A3 centre (136.1, 11.2) radius 43.6198
  line L11 (5.1, 54.8198) -> (149.8881, 54.8198)
  line L12 (75.6, 22.4) -> (65.6, 22.4) projected
  line L13 (70.6, 22.4) -> (70.6, 32.4)
  line L14 (70.6, 32.4) -> (43.2215, 32.4)
  line L15 (70.6, 32.4) -> (97.9785, 32.4)
  line L16 (136.1, 11.2) -> (169.1, 11.2)
  point P0 (-4.4, 0)
  point P1 (136.1, 54.8198)
  dimension "d128" = 66
  dimension "d124" = 16.2
  dimension "d125" = 20.5
  dimension "d126" = 20.5
  dimension "d127" = 66
  dimension "d129" = 25
  dimension "d130" = 50
  dimension "d131" = 10
  constraints: 24 end point, 6 point on line, 5 midpoint, 5 point on circle, 4 coincident, 3 centre point, 2 tangent, 1 horizontal, 1 horizontal alignment, 1 perpendicular, 1 vertical, 2 other
  measures "d124" distance of L0.start L4.end
  measures "d125" distance of L4.end L7.end
  measures "d126" distance of L6.end L8.end
  measures "d127" diameter of A0
  measures "d129" distance of L9.start L9.end
  measures "d130" distance of L9.end L10.end
  measures "d131" distance of L13.start L13.end
extrude "Extrusion31" add sketch "Sketch30" along normal blind 3 contours A2 L6 A3 L0 | A2 L14 L15 A3 L6
extrude "Extrusion32" add sketch "Sketch30" along normal blind 25 contours L11 A3 L15 L14 A2
chamfer "Chamfer1" distance 22 angle 45 1 edges at (75, 32.4, 27)
sketch "Sketch31" plane through (4.4, 0, -85.8) normal (0, 0, -1) x (-1, 0, 0)
  line L0 (-156.6, -5) -> (-156.6, 22.4) projected
  line L1 (-156.6, -5) -> (-156.6, 11.2)
  line L2 (-156.6, 11.2) -> (72.2154, 11.2)
  line L3 (-156.6, 11.2) -> (-136.1, 11.2)
  circle A0 centre (-136.1, 11.2) radius 33
  line L4 (-156.6, -5) -> (15.4, -5) projected
  line L5 (-70.6, -5) -> (-70.6, 49.7286)
  circle A1 centre (-136.1, 11.2) radius 43.62
  circle A2 centre (-5.1, 11.2) radius 33
  circle A3 centre (-5.1, 11.2) radius 43.62
  line L6 (-70.6, 22.3643) -> (-70.6, 32.3643)
  line L7 (-95.5998, -5) -> (-45.6002, -5)
  line L8 (-70.6, 32.3643) -> (-97.9585, 32.3643)
  line L9 (-70.6, 32.3643) -> (-43.2415, 32.3643)
  line L10 (-136.1, 54.82) -> (-5.1, 54.82)
  point P0 (4.4, 0)
  dimension "d139" = 16.2
  dimension "d140" = 90
  dimension "d141" = 20.5
  dimension "d142" = 66
  dimension "d143" = 87.24
  dimension "d144" = 10
  constraints: 18 end point, 6 point on circle, 6 point on line, 4 centre point, 3 coincident, 2 midpoint, 2 symmetric about line, 1 horizontal, 1 tangent, 1 vertical, 2 other
  measures "d139" distance of L0.start L1.end
  measures "d140" angle of L1 L2
  measures "d141" distance of L1.end L3.end
  measures "d142" diameter of A0
  measures "d143" diameter of A1
  measures "d144" distance of L6.start L6.end
extrude "Extrusion33" add sketch "Sketch31" along normal blind 3 contours A1 L2 L5 L4 | A1 L8 L5 L2 | L5 L2 A3 L4 | L5 L9 A3 L2
extrude "Extrusion34" add sketch "Sketch31" along normal blind 25 contours L10 A3 L9 L8 A1
chamfer "Chamfer2" distance 22 angle 45 1 edges at (75, 32.3643, -110.8)
sketch "Sketch32" plane through (9.5, 54.8198, 2) normal (0, 1, 0) x (1, 0, 0)
  line L0 (131, 0) -> (131, -25) projected
  line L1 (0, 87.8) -> (0, 112.8) projected
  line L2 (131, -25) -> (0, -25)
  line L3 (0, -25) -> (0, 112.8)
  line L4 (0, 112.8) -> (131, 112.8)
  line L5 (131, 112.8) -> (131, -25)
  line L6 (131, -25) -> (0, -25)
  line L7 (0, -25) -> (0, 0)
  line L8 (0, 0) -> (131, 0)
  line L9 (131, 0) -> (131, -25)
  line L10 (0, 87.8) -> (131, 87.8)
  line L11 (131, 87.8) -> (131, 112.8)
  line L12 (131, 112.8) -> (0, 112.8)
  line L13 (0, 112.8) -> (0, 87.8)
  line L14 (131, -25) -> (101, -25)
  line L15 (101, -25) -> (101, 0)
  line L16 (101, 0) -> (131, 0)
  line L17 (131, 0) -> (131, -25)
  line L18 (0, -25) -> (30, -25)
  line L19 (30, -25) -> (30, 0)
  line L20 (30, 0) -> (0, 0)
  line L21 (0, 0) -> (0, -25)
  circle A0 centre (101, -12.5) radius 2.7
  circle A1 centre (30, -12.5) radius 2.7
  line L22 (131, 100.3) -> (0, 100.3)
  line L23 (131, 43.9) -> (-33.0884, 43.9)
  circle A2 centre (101, 100.3) radius 2.7
  circle A3 centre (30, 100.3) radius 2.7
  point P0 (-9.5, 2)
  dimension "d152" = 30
  dimension "d153" = 30
  dimension "d154" = 5.4
  dimension "d155" = 5.4
  constraints: 44 end point, 10 parallel, 6 horizontal, 5 midpoint, 5 perpendicular, 4 centre point, 3 point on line, 2 symmetric about line, 2 other
  measures "d152" distance of L15.end L16.end
  measures "d153" distance of L20.end L19.end
  measures "d154" diameter of A0
  measures "d155" diameter of A1
extrude "Extrusion35" cut sketch "Sketch32" against normal blind 6 contours A0 L15 | L15 A0 | A1 L19 | L19 A1 | A2 L22 | L22 A2 | A3 L22 | L22 A3
sketch "Sketch33" plane through (9.5, 54.82, -85.8) normal (0, 1, 0) x (1, 0, 0)
  line L0 (87.38, 0) -> (131, 0) projected
  line L1 (0, 25) -> (131, 25) projected
  line L2 (131, 0) -> (0, 0)
  line L3 (0, 0) -> (0, 25)
  line L4 (0, 25) -> (131, 25)
  line L5 (131, 25) -> (131, 0)
  circle A0 centre (101, 12.5) radius 2.7 projected
  circle A1 centre (101, 12.5) radius 2.7
  circle A2 centre (30, 12.5) radius 2.7 projected
  circle A3 centre (30, 12.5) radius 2.7
  point P0 (-9.5, -85.8)
  point P1 (88.8424, 0)
  constraints: 8 end point, 2 centre point, 2 coincident, 2 parallel, 1 horizontal, 1 perpendicular
extrude "Extrusion36" cut sketch "Sketch33" against normal blind 6 contours A0 | A2
sketch "Sketch34" plane through (4.4, 0, 5) normal (0, 0, 1) x (1, 0, 0)
  line L0 (95.5998, -5) -> (45.6002, -5) projected
  line L1 (70.6, -5) -> (63.5, -5)
  line L2 (63.5, -5) -> (77.7, -5)
  line L3 (63.5, -5) -> (77.7, -5)
  line L4 (77.7, -5) -> (77.7, 26)
  line L5 (77.7, 26) -> (63.5, 26)
  line L6 (63.5, 26) -> (63.5, -5)
  line L7 (78.2, 26.5) -> (78.2, -5.5)
  line L8 (78.2, -5.5) -> (63, -5.5)
  line L9 (63, -5.5) -> (63, 26.5)
  line L10 (63, 26.5) -> (78.2, 26.5)
  point P0 (-4.4, 0)
  point P1 (78.2, -5)
  point P2 (63, -5)
  dimension "d160" = 7.1
  dimension "d161" = 14.2
  dimension "d162" = 31
  dimension "d163" = 0.5
  constraints: 20 end point, 4 parallel, 2 perpendicular, 2 point on line, 1 horizontal, 1 midpoint, 3 other
  measures "d160" distance of L1.start L1.end
  measures "d161" distance of L1.end L2.end
  measures "d162" distance of L4.end L3.end
  measures "d163" distance between parallel lines of L4 L7
extrude "Extrusion37" cut sketch "Sketch34" against normal blind 1.5 contours L4 L5 L6 L0 L9 L10 L7 | L0 L6 L5 L4
sketch "Sketch35" plane through (4.4, 0, 3.5) normal (0, 0, 1) x (1, 0, 0)
  line L0 (63, 26.5) -> (78.2, 26.5) projected
  line L1 (78.2, 26.5) -> (78.2, -5) projected
  line L2 (63, 26.5) -> (78.2, 26.5)
  line L3 (78.2, 26.5) -> (78.2, 21.5)
  line L4 (78.2, 21.5) -> (63, 21.5)
  line L5 (63, 21.5) -> (63, 26.5)
  point P0 (-4.4, 0)
  dimension "d166" = 5
  constraints: 8 end point, 2 parallel, 1 horizontal, 1 perpendicular, 1 point on line
  measures "d166" distance of L2.end L3.end
extrude "Extrusion38" cut sketch "Sketch35" against normal blind 1.25
sketch "Sketch36" plane through (4.4, 0, 3.5) normal (0, 0, 1) x (1, 0, 0)
  point P0 (-4.4, 0)
sketch "Sketch37" plane through (4.4, 0, -88.8) normal (0, 0, -1) x (-1, 0, 0)
  line L0 (-78.2, -5) -> (-63, -5) projected
  line L1 (-70.6, -5) -> (-78.2, -5)
  line L2 (-78.2, -5) -> (-63, -5)
  line L3 (-78.2, -5) -> (-95.6, -5) projected
  line L4 (-63, -5) -> (-63, 26.5) projected
  line L5 (-78.2, -5) -> (-63, -5)
  line L6 (-63, -5) -> (-63, 26.5)
  line L7 (-63, 26.5) -> (-78.2, 26.5)
  line L8 (-78.2, 26.5) -> (-78.2, -5)
  point P0 (4.4, 0)
  dimension "d169" = 7.6
  dimension "d170" = 15.2
  constraints: 12 end point, 2 collinear, 2 parallel, 1 horizontal, 1 midpoint, 1 perpendicular
  measures "d169" distance of L1.start L0.start
  measures "d170" distance of L0.start L0.end
extrude "Extrusion39" cut sketch "Sketch37" against normal blind 1.5
sketch "Sketch38" plane through (4.4, 0, -87.3) normal (0, 0, -1) x (-1, 0, 0)
  line L0 (-63, 26.5) -> (-78.2, 26.5) projected
  line L1 (-78.2, 21.5) -> (-63, 21.5) projected
  line L2 (-78.2, 26.5) -> (-63, 26.5)
  line L3 (-63, 26.5) -> (-63, 21.5)
  line L4 (-63, 21.5) -> (-78.2, 21.5)
  line L5 (-78.2, 21.5) -> (-78.2, 26.5)
  point P0 (4.4, 0)
  constraints: 8 end point, 2 parallel, 1 horizontal, 1 perpendicular
extrude "Extrusion40" cut sketch "Sketch38" against normal blind 1.25
sketch "Sketch39" plane through (4.4, 0, -87.3) normal (0, 0, -1) x (-1, 0, 0)
  line L0 (-63, 21.5) -> (-63, 26.5) projected
  line L1 (-63, 26.5) -> (-63, 19)
  line L2 (-63, 26.5) -> (-78.2, 26.5) projected
  line L3 (-70.6, 26.5) -> (-70.6, 16.4)
  line L4 (-73.3, 16.4) -> (-67.9, 16.4) projected
  line L5 (-70.6, 19) -> (-63, 19)
  circle A0 centre (-70.6, 19) radius 2.05
  point P0 (4.4, 0)
  dimension "d175" = 7.5
  dimension "d176" = 4.1
  constraints: 6 end point, 2 midpoint, 1 centre point, 1 coincident, 1 horizontal, 1 point on line, 1 vertical
  measures "d175" distance of L0.end L1.end
  measures "d176" diameter of A0
extrude "Extrusion41" cut sketch "Sketch39" against normal through all contours A0 L3 L5 | L5 L3 A0 | L3 A0
sketch "Sketch40" plane through (4.4, 0, -86.05) normal (0, 0, -1) x (-1, 0, 0)
  line L0 (-63, 26.5) -> (-78.2, 26.5) projected
  line L1 (-78.2, 21.5) -> (-63, 21.5) projected
  line L2 (-78.2, 26.5) -> (-63, 26.5)
  line L3 (-63, 26.5) -> (-63, 21.5)
  line L4 (-63, 21.5) -> (-78.2, 21.5)
  line L5 (-78.2, 21.5) -> (-78.2, 26.5)
  point P0 (4.4, 0)
  constraints: 8 end point, 2 parallel, 1 horizontal, 1 perpendicular
extrude "Extrusion42" cut sketch "Sketch40" against normal through all
sketch "Sketch41" plane through (0, 0, 0) normal (0, 1, 0) x (1, 0, 0)
  line L0 (70, -2) -> (70, 85.8) projected
  line L1 (70, 41.9) -> (70, 49)
  line L2 (70, 49) -> (70, 34.8)
  line L3 (70, 49) -> (70, 49.25)
  line L4 (70, 34.8) -> (70, 34.55)
  line L5 (70, 34.55) -> (70, 49.25)
  line L6 (70, 49.25) -> (62.5, 49.25)
  line L7 (62.5, 49.25) -> (62.5, 34.55)
  line L8 (62.5, 34.55) -> (70, 34.55)
  line L9 (70, 34.55) -> (70, 49.25)
  point P0 (0, 0)
  dimension "d181" = 7.1
  dimension "d182" = 14.2
  dimension "d183" = 0.25
  dimension "d184" = 0.25
  dimension "d185" = 7.5
  constraints: 18 end point, 4 point on line, 2 parallel, 1 collinear, 1 horizontal, 1 midpoint, 1 perpendicular
  measures "d181" distance of L1.start L1.end
  measures "d182" distance of L1.end L2.end
  measures "d183" distance of L1.end L3.end
  measures "d184" distance of L2.end L4.end
  measures "d185" distance of L8.end L7.end
extrude "Extrusion43" cut sketch "Sketch41" against normal blind 10
sketch "Sketch42" plane through (70, 11.2, -11.2) normal (-1, 0, 0) x (0, 0, 1)
  line L0 (-23.35, -16.2) -> (-38.05, -16.2) projected
  line L1 (-38.05, -16.2) -> (-38.05, 14.8)
  line L2 (-38.05, 14.8) -> (-23.35, 14.8)
  line L3 (-23.35, 14.8) -> (-23.35, -16.2)
  line L4 (-23.35, -16.2) -> (-38.05, -16.2)
  line L5 (-38.05, -16.2) -> (-38.05, 14.8)
  line L6 (-30.7, 14.8) -> (-30.7, -0.2)
  circle A0 centre (-30.7, -0.2) radius 2
  point P0 (11.2, -11.2)
  dimension "d188" = 31
  dimension "d189" = 15
  dimension "d190" = 4
  constraints: 12 end point, 2 parallel, 2 vertical, 1 centre point, 1 coincident, 1 horizontal, 1 midpoint, 1 perpendicular
  measures "d188" distance of L0.end L1.end
  measures "d189" distance of L6.start L6.end
  measures "d190" diameter of A0
extrude "Extrusion44" cut sketch "Sketch42" against normal blind 10 contours A0
sketch "Sketch43" plane through (80, 0, -13.2) normal (1, 0, 0) x (0, 0, -1)
  circle A0 centre (28.7, 11) radius 2 projected
  circle A1 centre (28.7, 11) radius 2.75
  point P0 (-13.2, 0)
  dimension "d193" = 5.5
  constraints: 1 centre point, 1 coincident
  measures "d193" diameter of A1
extrude "Extrusion45" cut sketch "Sketch43" against normal up to surface (10 mm away) contours A0 | A1
sketch "Sketch44" plane through (108, 22.4, -24.4) normal (0, 1, 0) x (1, 0, 0)
  line L0 (0, 40) -> (19.6, 40) projected
  line L1 (53, 61.4) -> (53, -26.4) projected
  line L2 (0, 40) -> (53, 40)
  line L3 (53, 40) -> (53, -5)
  line L4 (53, -5) -> (0, -5)
  line L5 (0, -5) -> (0, 40)
  point P0 (-108, -24.4)
  dimension "d196" = 45
  dimension "d197" = 53
  constraints: 8 end point, 2 parallel, 1 horizontal, 1 perpendicular, 1 point on line
  measures "d196" distance of L2.end L3.end
  measures "d197" distance of L0.start L2.end
sketch "Sketch45" plane through (4.4, 0, -85.8) normal (0, 0, 1) x (1, 0, 0)
  arc A0 (47.2576, 0) -> (5.1, 54.82) centre (5.1, 11.2) ccw projected
  line L0 (5.1, 54.82) -> (136.1, 54.82)
  line L1 (136.1, 54.82) -> (136.1, 26.5)
  line L2 (136.1, 26.5) -> (5.1, 26.5)
  line L3 (5.1, 26.5) -> (5.1, 54.82)
  point P0 (-4.4, 0)
  point P1 (45.9487, 26.5)
  dimension "d198" = 131
  constraints: 8 end point, 2 parallel, 1 horizontal, 1 perpendicular
  measures "d198" distance of L1.end L2.end
extrude "Extrusion46" cut sketch "Sketch45" against normal blind 40 contours A0 L0 L1 L2
sketch "Sketch46" plane through (4.4, 0, 2) normal (0, 0, -1) x (-1, 0, 0)
  line L0 (-136.1, 54.8198) -> (-5.1, 54.8198) projected
  arc A0 (-45.9487, 26.5) -> (-45.6002, -5) centre (-5.1, 11.2) ccw projected
  line L1 (-136.1, 54.8198) -> (-45.9487, 54.8198)
  line L2 (-45.9487, 54.8198) -> (-45.9487, 26.5)
  line L3 (-45.9487, 26.5) -> (-136.1, 26.5)
  line L4 (-136.1, 26.5) -> (-136.1, 54.8198)
  line L5 (-45.9487, 26.5) -> (8.4354, 26.5)
  line L6 (8.4354, 26.5) -> (8.4354, 61.3657)
  line L7 (8.4354, 61.3657) -> (-45.9487, 61.3657)
  line L8 (-45.9487, 61.3657) -> (-45.9487, 26.5)
  point P0 (4.4, 0)
  point P1 (-45.9487, 54.8198)
  constraints: 16 end point, 4 parallel, 2 horizontal, 2 perpendicular
extrude "Extrusion47" cut sketch "Sketch46" against normal blind 40
sketch "Sketch47" plane through (4.4, 0, 3.5) normal (0, 0, 1) x (1, 0, 0)
  line L0 (63, 21.5) -> (78.2, 21.5)
  line L1 (78.2, 21.5) -> (78.2, -5)
  line L2 (78.2, -5) -> (63, -5)
  line L3 (63, -5) -> (63, 21.5)
  circle A0 centre (70.6, 19) radius 2.05 projected
  circle A1 centre (70.6, 19) radius 2.05
  line L4 (-15.4, -5) -> (45.6, -5) projected
  line L5 (70.6, -5) -> (-15.4, -5)
  line L6 (-15.4, -5) -> (-0.2, -5)
  line L7 (-0.2, -5) -> (-0.2, 21.5)
  line L8 (-0.2, 21.5) -> (-15.4, 21.5)
  line L9 (-15.4, 21.5) -> (-15.4, -5)
  line L10 (-15.4, 21.5) -> (-0.2, 21.5)
  line L11 (-0.2, 21.5) -> (-0.2, 19)
  line L12 (-0.2, 19) -> (-15.4, 19)
  line L13 (-15.4, 19) -> (-15.4, 21.5)
  circle A2 centre (-7.8, 19) radius 2.05
  point P0 (-4.4, 0)
  dimension "d203" = 2.5
  dimension "d204" = 15.2
  dimension "d205" = 26.5
  dimension "d206" = 15.2
  dimension "d207" = 26.5
  dimension "d208" = 2.5
  dimension "d209" = 4.1
  constraints: 26 end point, 6 parallel, 3 horizontal, 3 perpendicular, 2 centre point, 2 midpoint, 1 coincident, 1 collinear, 1 point on line
  measures "d203" distance from line of L0 A1.centre
  measures "d204" distance of L1.end L2.end
  measures "d205" distance of L2.end L0.start
  measures "d206" distance of L8.end L7.end
  measures "d207" distance of L7.end L6.end
  measures "d208" distance of L10.end L11.end
  measures "d209" diameter of A2
extrude "Extrusion48" add sketch "Sketch47" against normal through all contours A2 L12 | L12 A2
sketch "Sketch48" plane through (-3.4, 19, 3.5) normal (0, 0, 1) x (1, 0, 0)
  circle A0 centre (0, 0) radius 2.05
  point P0 (3.4, -19)
  constraints: 1 centre point
extrude "Extrusion49" cut sketch "Sketch48" against normal through all
sketch "Sketch49" plane through (4.4, 0, 2) normal (0, 0, 1) x (1, 0, 0)
  circle A0 centre (-7.8, 19) radius 2.05 projected
  circle A1 centre (-7.8, 19) radius 2.15
  point P0 (-4.4, 0)
  dimension "d214" = 4.3
  constraints: 1 centre point, 1 coincident
  measures "d214" diameter of A1
extrude "Extrusion50" cut sketch "Sketch49" against normal through all
body "Solid1"
